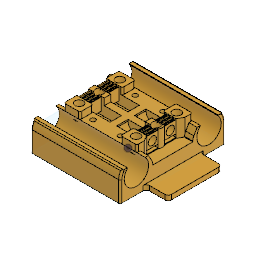
Direct_X_carriage v7 (Autodesk Fusion 360 design; units mm, degrees)
Autodesk Fusion 360 part; units mm, degrees
note: some values were not read from the file. Set by a fixed rule: which face or edge a step refers to.
sketch "スケッチ1" plane through (0, 0, 0) normal (0, 0, 1) x (1, 0, 0)
  line L0 (-27.5, 32.3) -> (27.5, 32.3)
  line L1 (27.5, 32.3) -> (27.5, 12.3)
  line L2 (27.5, 12.3) -> (18.5, 12.3)
  line L3 (18.5, 12.3) -> (18.5, -12.3)
  line L4 (18.5, -12.3) -> (27.5, -12.3)
  line L5 (27.5, -12.3) -> (27.5, -32.3)
  line L6 (27.5, -32.3) -> (-27.5, -32.3)
  line L7 (-27.5, -32.3) -> (-27.5, -12.3)
  line L8 (-27.5, -12.3) -> (-18.5, -12.3)
  line L9 (-18.5, -12.3) -> (-18.5, 12.3)
  line L10 (-18.5, 12.3) -> (-27.5, 12.3)
  line L11 (-27.5, 12.3) -> (-27.5, 32.3)
  circle A0 centre (0, 0) radius 1.75
  dimension "d1" = 55
  dimension "d2" = 64.6
  dimension "d3" = 20
  dimension "d4" = 20
  dimension "d5" = 9
  dimension "d6" = 27.5
  dimension "d7" = 32.3
  dimension "d8" = 9
  dimension "d9" = 3.5
  constraint perpendicular L0 L1
  constraint perpendicular L1 L2
  constraint perpendicular L2 L3
  constraint perpendicular L1 L4
  constraint perpendicular L4 L5
  constraint perpendicular L5 L6
  constraint perpendicular L4 L7
  constraint perpendicular L7 L8
  constraint perpendicular L8 L9
  constraint perpendicular L9 L10
  constraint perpendicular L0 L11
  constraint collinear L2 L10
  constraint collinear L4 L8
  constraint collinear L1 L5
  constraint collinear L7 L11
  constraint horizontal L0
  constraint coincident A0.centre origin
  measures "d1" horizontal distance of L5.end L6.end
  measures "d2" distance of L0 L6
  measures "d3" vertical distance of L0.end L1.end
  measures "d4" vertical distance of L4.end L5.end
  measures "d5" horizontal distance of L1.end L2.end
  measures "d6" distance of A0.centre L5
  measures "d7" distance of A0.centre L0
  measures "d8" horizontal distance of L9.end L10.end
  measures "d9" diameter of A0
extrude "押し出し1" add sketch "スケッチ1" along normal blind 17.3 makes body 1
sketch "スケッチ2" plane through (27.5, 0, 0) normal (1, 0, 0) x (0, 1, 0)
  line L0 (12.3, 0) -> (32.3, 0)
  line L1 (32.3, 0) -> (32.3, 17.3)
  line L2 (32.3, 17.3) -> (12.3, 17.3)
  line L3 (12.3, 17.3) -> (12.3, 0)
  line L4 (22.3, 0) -> (22.3, 17.3) construction
  line L5 (12.3, 12.6228) -> (32.3, 12.6228) construction
  circle A0 centre (22.3, 12) radius 7.495
  line L6 (32.3, 12.6228) -> (29.5996, 17.3)
  line L7 (32.3, 12.6228) -> (38.6199, 12.6228) construction
  line L8 (12.3, 12.6228) -> (15.0004, 17.3)
  line L9 (12.3, 17.3) -> (-12.3, 17.3)
  line L10 (0, 0) -> (0, 17.3) construction
  circle A1 centre (-22.3, 12) radius 7.495
  line L11 (-12.3, 12.6228) -> (-15.0004, 17.3)
  line L12 (-32.3, 12.6228) -> (-29.5996, 17.3)
  line L13 (-32.3, 17.3) -> (-12.3, 17.3)
  line L14 (-32.3, 0) -> (-32.3, 17.3)
  line L15 (-12.3, 17.3) -> (-12.3, 0)
  circle A2 centre (22.3, 12) radius 10.0194
  circle A3 centre (-22.3, 12) radius 10.0194
  point P0 (0, 17.3)
  dimension "d12" = 12.6228
  dimension "d13" = 14.99
  dimension "d14" = 120
  dimension "d15" = 60
  dimension "d135" = 12
  constraint midpoint L0 L4.start
  constraint midpoint L2 L4.end
  constraint coincident L3 L5.start
  constraint coincident L1 L5.end
  constraint perpendicular L1 L5
  constraint coincident L2 L6.end
  constraint horizontal L7
  constraint coincident L2 L8.end
  constraint coincident L4 A0.centre
  constraint coincident L10.start origin
  constraint coincident P0 L10.end
  constraint symmetric L5.start L10 L11.start
  constraint symmetric L5.end L10 L12.start
  constraint symmetric A0 L10 A1
  constraint symmetric L6.end L10 L12.end
  constraint symmetric L8.end L10 L11.end
  constraint symmetric L0.start L10 L15.end
  constraint symmetric L0.end L10 L14.start
  constraint symmetric L1.end L10 L13.start
  constraint symmetric L2.end L10 L9.end
  constraint concentric A0 A2
  constraint coincident L5.end A2
  constraint concentric A1 A3
  constraint coincident L12.start A3
  measures "d12" distance of L0 L5
  measures "d13" diameter of A0
  measures "d14" angle of L6 L7
  measures "d15" angle of L7 L8
  measures "d135" distance of L4.start A0.centre
extrude "押し出し2" cut sketch "スケッチ2" against normal blind 55 contours L1 L2 A2 | L2 A0 | A1 L13 | L13 L14 A3 picked at (23.4851, 8.0373) picked at (-20.2164, 11.6826) bodies 1
extrude "押し出し3" cut sketch "スケッチ2" against normal blind 9 contours L2 L8 A2 | L2 L3 A2 | L11 L13 A3 | L13 L15 A3 bodies 1
extrude "押し出し4" cut sketch "スケッチ2" against normal blind 9 from surface at -46 contours L2 L8 A2 | L2 L3 A2 | L11 L13 A3 | L13 L15 A3 bodies 1
sketch "スケッチ3" plane through (0, 0, 17.3) normal (0, 0, 1) x (-1, 0, 0)
  line L0 (18.5, -15.0004) -> (18.5, 15.0004)
  line L1 (27.5, 15.0004) -> (27.5, 17.0005)
  line L2 (-27.5, 17.0005) -> (-27.5, 15.0004)
  line L3 (-18.5, 15.0004) -> (-18.5, -15.0004)
  line L4 (-18.5, -15.0004) -> (-27.5, -15.0004)
  line L5 (-27.5, -15.0004) -> (-27.5, -17.0005)
  line L6 (-27.5, -17.0005) -> (27.5, -17.0005)
  line L7 (27.5, -17.0005) -> (27.5, -15.0004)
  line L8 (27.5, -15.0004) -> (18.5, -15.0004)
  circle A0 centre (0, 0) radius 1.75
  line L9 (-12.5, -17.0005) -> (-12.5, -9)
  line L10 (-2, -9) -> (-22.5, -9)
  line L11 (-22.5, -9) -> (-22.5, -17.0005)
  line L12 (-22.5, -17.0005) -> (-12.5, -17.0005)
  line L13 (-2, -9) -> (-2, -2)
  line L14 (-2, -2) -> (-18.5, -2)
  line L15 (27.5, 17.0005) -> (-27.5, 17.0005)
  line L16 (-27.5, 15.0004) -> (-18.5, 15.0004)
  line L17 (18.5, 15.0004) -> (27.5, 15.0004)
  dimension "d23" = 10
  dimension "d24" = 12.5
  dimension "d26" = 7
  dimension "d27" = 2
  dimension "d28" = 16.5
  constraint coincident L6 L9.start
  constraint perpendicular L6 L9
  constraint perpendicular L9 L10
  constraint coincident L6 L11.end
  constraint perpendicular L6 L11
  constraint vertical L13
  constraint coincident L3 L14.end
  constraint perpendicular L3 L14
  constraint coincident L9.end L10
  measures "d23" horizontal distance of L9.start L11.end
  measures "d24" horizontal distance of A0.centre L9.start
  measures "d26" vertical distance of L13.end L10.start
  measures "d27" distance of A0.centre L14
  measures "d28" horizontal distance of L13.end L14.end
extrude "押し出し5" cut sketch "スケッチ3" against normal blind 5.9 contours L3 L10 L13 L14 bodies 1
fillet "フィレット3" radius 5 1 edges at (2, 5.5, 11.4) on bodies 1
mirror "ミラー1" about plane through (0, 0, 0) normal (0, 1, 0) of "押し出し5", "フィレット3"
mirror "ミラー2" about plane through (0, 0, 0) normal (1, 0, 0) of "押し出し5", "フィレット3", "ミラー1"
extrude "押し出し6" add sketch "スケッチ3" against normal blind 12.3 separate body contours L3 L4 L6 L9 L10 L11 L12 | L3 L4 L10 L11 makes body 2
chamfer "面取り2" distance 4 distance2 6.4 1 edges at (22.5, 13.0002, 5) measured on face at (17.8333, 13.667, 5) on bodies 2
extrude "押し出し7" add sketch "スケッチ3" along normal blind 4.1 contours L3 L4 L6 L9 L10 L11 L12 | L3 L4 L10 L11 bodies 2
chamfer "面取り3" distance 2 distance2 3.5 1 edges at (22.5, 9, 16.4) measured on face at (15.8333, 9, 12.6) on bodies 2
sketch "スケッチ4" plane through (0, 0, 21.4) normal (0, 0, 1) x (-1, 0, 0)
  line L0 (-20.5, -9) -> (-22.5, -12.5)
  line L1 (-22.5, -12.5) -> (-22.5, -17.0005)
  line L2 (-22.5, -17.0005) -> (-12.5, -17.0005)
  line L3 (-12.5, -17.0005) -> (-12.5, -9)
  line L4 (-12.5, -9) -> (-20.5, -9)
  line L5 (-17.5, -9) -> (-17.5, -17.0005) construction
  line L6 (-22.5, -12.5) -> (-12.5, -12.5) construction
  circle A0 centre (-17.5, -12.5) radius 1.75
  circle A1 centre (-17.5, -12.5) radius 2.35
  circle A2 centre (-17.5, -12.5) radius 2.5
  dimension "d47" = 3.5
  dimension "d48" = 5
  dimension "d50" = 5
  dimension "d51" = 4.7
  dimension "d53" = 3.5
  constraint coincident L4 L5.start
  constraint coincident L2 L5.end
  constraint coincident L1 L0.end
  constraint coincident L3 L6.end
  constraint perpendicular L4 L5
  constraint perpendicular L3 L6
  constraint midpoint L6 A0.centre
  constraint concentric A0 A1
  constraint concentric A1 A2
  measures "d47" distance of L3.end L6.end
  measures "d48" distance of L1 L5
  measures "d50" diameter of A2
  measures "d51" diameter of A1
  measures "d53" diameter of A0
fillet "フィレット1" radius 1 3 edges at (12.5, 9, 13.2) (12.5, 17.0005, 13.2) (22.5, 17.0005, 16.4) on bodies 2
extrude "押し出し19" cut sketch "スケッチ2" against normal blind 20 contours L2 A0 picked at (23.4851, 8.0373) bodies 2
mirror "ミラー3" about plane through (0, 0, 0) normal (0, 1, 0) of bodies 2 makes body 3
sketch "スケッチ5" plane through (0, 9, 0) normal (0, -1, 0) x (1, 0, 0)
  line L0 (13.5, 21.4) -> (13.5, 5)
  line L1 (13.5, 5) -> (18.5, 5)
  line L2 (18.5, 5) -> (20.5, 8.2)
  line L3 (20.5, 8.2) -> (20.5, 21.4)
  line L4 (20.5, 21.4) -> (13.5, 21.4)
  line L5 (13.5, 13.4) -> (20.5, 13.4)
  line L6 (14.5, 13.4) -> (14.5, 21.4)
  line L7 (20.5, 20.95) -> (14.5, 20.95)
  line L8 (17.5, 20.95) -> (17.5, 20.2) construction
  arc A0 (17.0011, 20.5118) -> (17.9989, 20.5118) centre (17.5, 20.755) ccw
  arc A1 (16.9, 20.95) -> (17.0011, 20.5118) centre (17.9, 20.95) ccw
  arc A2 (17.9989, 20.5118) -> (18.1, 20.95) centre (17.1, 20.95) ccw
  arc A3 (15.9989, 20.5118) -> (16.1, 20.95) centre (15.1, 20.95) ccw
  arc A4 (15.0011, 20.5118) -> (15.9989, 20.5118) centre (15.5, 20.755) ccw
  arc A5 (14.9, 20.95) -> (15.0011, 20.5118) centre (15.9, 20.95) ccw
  arc A6 (19.9989, 20.5118) -> (20.1, 20.95) centre (19.1, 20.95) ccw
  arc A7 (19.0011, 20.5118) -> (19.9989, 20.5118) centre (19.5, 20.755) ccw
  arc A8 (18.9, 20.95) -> (19.0011, 20.5118) centre (19.9, 20.95) ccw
  dimension "d62" = 8
  dimension "d63" = 6
  dimension "d64" = 0.45
  dimension "d65" = 0.75
  dimension "d70" = 0.555
  dimension "d71" = 1
  dimension "d72" = 1
  dimension "d75" = 2
  dimension "d76" = 0
  constraint coincident L0 L5.start
  constraint coincident L3 L5.end
  constraint perpendicular L0 L5
  constraint coincident L5 L6.start
  constraint coincident L4 L6.end
  constraint perpendicular L5 L6
  constraint coincident L3 L7.start
  constraint coincident L6 L7.end
  constraint perpendicular L6 L7
  constraint midpoint L7 L8.start
  constraint vertical L8
  constraint coincident L8 A0.centre
  constraint coincident L7 A1.centre
  constraint coincident L7 A2.centre
  constraint coincident L7 A1.start
  constraint coincident L7 A2.end
  constraint coincident L8.end A0
  constraint tangent A0 A1
  constraint coincident A0.start A1.end
  constraint coincident A0.end A2.start
  constraint tangent A0 A2
  measures "d62" distance of L4 L5
  measures "d63" distance of L3 L6
  measures "d64" distance of L4 L7
  measures "d65" distance of L8.start L8.end
  measures "d70" radius of A0
  measures "d71" radius of A1
  measures "d72" radius of A2
extrude "押し出し11" add sketch "スケッチ5" along normal up to surface (18 mm away) contours L3 L5 L6 L7 A0 A1 A2 A3 A4 A5 A6 A7 A8 bodies 2 3
fillet "フィレット2" radius 0.0001 6 edges at (14.9, 0, 20.95) (16.1, 0, 20.95) (16.9, 0, 20.95) (18.1, 0, 20.95) (18.9, 0, 20.95) (20.1, 0, 20.95) on bodies 2
sketch "スケッチ6" plane through (0, 0, 13.4) normal (0, 0, -1) x (1, 0, 0)
  line L0 (20.5, 9) -> (14.5, 9)
  line L1 (14.5, 9) -> (14.5, -9)
  line L2 (14.5, -9) -> (20.5, -9)
  line L3 (20.5, -9) -> (20.5, 9)
  line L4 (14.5, 0) -> (20.5, 0) construction
  line L5 (14.5, 2) -> (20.5, 2)
  line L6 (14.5, -2) -> (20.5, -2)
  dimension "d87" = 2
  dimension "d88" = 2
  constraint midpoint L1 L4.start
  constraint midpoint L3 L4.end
  constraint coincident L1 L5.start
  constraint coincident L3 L5.end
  constraint perpendicular L3 L5
  constraint coincident L1 L6.start
  constraint coincident L3 L6.end
  constraint perpendicular L3 L6
  measures "d87" distance of L4 L5
  measures "d88" distance of L4 L6
extrude "押し出し15" add sketch "スケッチ6" against normal blind 8 contours L1 L3 L5 L6 bodies 2
sketch "スケッチ7" plane through (0, 0, 21.4) normal (0, 0, 1) x (-1, 0, 0)
  line L0 (-14.5, -2) -> (-14.5, 2)
  line L1 (-14.5, 2) -> (-20.5, 2)
  line L2 (-20.5, 2) -> (-20.5, -2)
  line L3 (-20.5, -2) -> (-14.5, -2)
  line L4 (-14.5, 0) -> (-20.5, 0) construction
  circle A0 centre (-17.5, 0) radius 2
  circle A1 centre (-17.5, 0) radius 2.5
  circle A2 centre (-17.5, 0) radius 2.55
  dimension "d91" = 4
  dimension "d92" = 5
  dimension "d93" = 5.1
  constraint midpoint L0 L4.start
  constraint midpoint L2 L4.end
  constraint midpoint L4 A0.centre
  constraint concentric A0 A1
  constraint concentric A1 A2
  measures "d91" diameter of A0
  measures "d92" diameter of A1
  measures "d93" diameter of A2
sketch "スケッチ8" plane through (20.5, 0, 0) normal (1, 0, 0) x (0, 1, 0)
  line L0 (-9, 13.4) -> (9, 13.4)
  line L1 (9, 13.4) -> (9, 20.95)
  line L2 (9, 20.95) -> (2, 20.95)
  line L3 (2, 20.95) -> (2, 21.4)
  line L4 (2, 21.4) -> (-2, 21.4)
  line L5 (-2, 21.4) -> (-2, 20.95)
  line L6 (-2, 20.95) -> (-9, 20.95)
  line L7 (-9, 20.95) -> (-9, 13.4)
  line L8 (9, 16.9) -> (-9, 16.9) construction
  line L9 (5.5, 13.4) -> (5.5, 20.95) construction
  circle A0 centre (5.5, 16.9) radius 2.55
  circle A1 centre (5.5, 16.9) radius 2.55
  dimension "d104" = 3.5
  dimension "d105" = 3.5
  dimension "d106" = 5.1
  dimension "d107" = 5.1
  constraint coincident L7 L8.end
  constraint coincident L0 L9.start
  constraint coincident L2 L9.end
  constraint perpendicular L2 L9
  constraint coincident L8 A0.centre
  constraint coincident L9 A0.centre
  constraint concentric A0 A1
  measures "d104" distance of L1 L9
  measures "d105" distance of L0 L8
  measures "d106" diameter of A0
  measures "d107" diameter of A1
extrude "押し出し20" cut sketch "スケッチ8" against normal blind 10 contours A0 A1 bodies 2
extrude "押し出し21" cut sketch "スケッチ8" against normal blind 0.5 contours A0 A1 bodies 2
mirror "ミラー6" about plane through (0, 0, 0) normal (0, 1, 0) of "押し出し20", "押し出し21"
mirror "ミラー5" about plane through (0, 0, 0) normal (1, 0, 0) of bodies 2 makes body 4
combine "結合1" operation add target body 1 tool bodies 2 4
sketch "スケッチ9" plane through (0, 0, 21.4) normal (0, 0, 1) x (-1, 0, 0)
  line L0 (-22.5, -12.5) -> (-22.5, -16.0005)
  arc A0 (-22.5, -16.0005) -> (-21.5, -17.0005) centre (-21.5, -16.0005) ccw
  line L1 (-21.5, -17.0005) -> (-13.5, -17.0005)
  arc A1 (-13.5, -17.0005) -> (-12.5, -16.0005) centre (-13.5, -16.0005) ccw
  line L2 (-12.5, -16.0005) -> (-12.5, -10)
  arc A2 (-12.5, -10) -> (-13.5, -9) centre (-13.5, -10) ccw
  line L3 (-13.5, -9) -> (-20.5, -9)
  line L4 (-20.5, -9) -> (-22.5, -12.5)
  line L5 (-12.5, -12.5) -> (-22.5, -12.5) construction
  line L6 (-17.5, -17.0005) -> (-17.5, -8.8071) construction
  circle A3 centre (-17.5, -12.5) radius 2
  circle A4 centre (-17.5, -12.5) radius 2.55
  circle A5 centre (-17.5, -12.5) radius 2.55
  dimension "d113" = 5
  dimension "d114" = 3.5
  dimension "d115" = 5.1
  dimension "d116" = 5.1
  dimension "d117" = 4
  constraint coincident L2 L5.start
  constraint coincident L0 L4.end
  constraint coincident L1 L6.start
  constraint perpendicular L1 L6
  constraint perpendicular L2 L5
  constraint midpoint L5 A3.centre
  constraint concentric A3 A4
  constraint concentric A4 A5
  measures "d113" distance of L2 L6
  measures "d114" distance of L3 L5
  measures "d115" diameter of A5
  measures "d116" diameter of A4
  measures "d117" diameter of A3
extrude "押し出し22" [suppressed]
extrude "押し出し23" cut sketch "スケッチ9" against normal blind 8 contours A3 | A4 A5 bodies 1
extrude "押し出し24" cut sketch "スケッチ9" against normal blind 0.5 contours A3 | A4 A5 bodies 1
mirror "ミラー7" about plane through (0, 0, 0) normal (0, 1, 0) of "押し出し23", "押し出し24"
mirror "ミラー8" about plane through (0, 0, 0) normal (1, 0, 0) of "押し出し23", "押し出し24", "ミラー7"
extrude "押し出し25" [suppressed]
extrude "押し出し26" cut sketch "スケッチ7" against normal blind 7 contours L3 A1 A2 | L1 L3 A1 A2 | L1 A1 A2 | L3 A1 | L1 L3 A0 A1 | L1 L3 A1 A2 | L1 A1 | L1 L3 A0 A1 | A0 bodies 1
extrude "押し出し27" [suppressed]
mirror "ミラー9" about plane through (0, 0, 0) normal (1, 0, 0) of "押し出し26"
fillet "フィレット4" radius 5 6 edges at (0, 32.3, 12.6228) (24.9429, 12.3, 12.6228) (-24.9429, 12.3, 12.6228) (0, -32.3, 12.6228) (24.9429, -12.3, 12.6228) (-24.9429, -12.3, 12.6228) on bodies 1
fillet "フィレット5" radius 1 10 edges at (27.5, 32.3, 6.3114) (-27.5, 32.3, 6.3114) (-27.5, -32.3, 6.3114) (27.5, -32.3, 6.3114) (27.5, 31.8424, 15.0546) (-27.5, 31.8424, 15.0546) (0, 30.8028, 17.3) (27.5, -31.8424, 15.0546) (-27.5, -31.8424, 15.0546) (0, -30.8028, 17.3) on bodies 1
chamfer "Chamfer6" distance 0.4 angle 45 2 edges at (0, -27.5995, 17.3) (0, 27.5995, 17.3) on bodies 1
sketch "スケッチ10" plane through (0, 0, 0) normal (0, 0, -1) x (1, 0, 0)
  circle A0 centre (0, 0) radius 1.75
  line L0 (27.5, 12.3) -> (27.5, 31.3)
  arc A1 (27.5, 31.3) -> (26.5, 32.3) centre (26.5, 31.3) ccw
  line L1 (26.5, 32.3) -> (-26.5, 32.3)
  arc A2 (-26.5, 32.3) -> (-27.5, 31.3) centre (-26.5, 31.3) ccw
  line L2 (-27.5, 31.3) -> (-27.5, 12.3)
  line L3 (-27.5, 12.3) -> (-18.5, 12.3)
  line L4 (-18.5, 12.3) -> (-18.5, -12.3)
  line L5 (-18.5, -12.3) -> (-27.5, -12.3)
  line L6 (-27.5, -12.3) -> (-27.5, -31.3)
  arc A3 (-27.5, -31.3) -> (-26.5, -32.3) centre (-26.5, -31.3) ccw
  line L7 (-26.5, -32.3) -> (26.5, -32.3)
  arc A4 (26.5, -32.3) -> (27.5, -31.3) centre (26.5, -31.3) ccw
  line L8 (27.5, -31.3) -> (27.5, -12.3)
  line L9 (27.5, -12.3) -> (18.5, -12.3)
  line L10 (18.5, -12.3) -> (18.5, 12.3)
  line L11 (18.5, 12.3) -> (27.5, 12.3)
  circle A5 centre (12, 12) radius 1.525
  circle A6 centre (-12, 12) radius 1.525
  circle A7 centre (-12, -12) radius 1.525
  circle A8 centre (12, -12) radius 1.525
  dimension "d139" = 3.05
  dimension "d140" = 12
  dimension "d141" = 12
  dimension "d143" = 360
  measures "d139" diameter of A5
  measures "d140" horizontal distance of A0.centre A5.centre
  measures "d141" vertical distance of A0.centre A5.centre
extrude "押し出し28" [suppressed]
sketch "Sketch39" plane through (0, 0, 17.3) normal (0, 0, 1) x (-1, 0, 0)
  circle A0 centre (0, 0) radius 1.75
  line L0 (14.5, -2) -> (14.5, 2)
  line L1 (14.5, 2) -> (2, 2)
  line L2 (2, 2) -> (2, 9)
  line L3 (2, 9) -> (13.5, 9)
  arc A1 (12.5, 10) -> (13.5, 9) centre (13.5, 10) ccw
  line L4 (12.5, 10) -> (12.5, 16.0005)
  arc A2 (13.5, 17.0005) -> (12.5, 16.0005) centre (13.5, 16.0005) ccw
  line L5 (13.5, 17.0005) -> (-13.5, 17.0005)
  arc A3 (-12.5, 16.0005) -> (-13.5, 17.0005) centre (-13.5, 16.0005) ccw
  line L6 (-12.5, 16.0005) -> (-12.5, 10)
  arc A4 (-13.5, 9) -> (-12.5, 10) centre (-13.5, 10) ccw
  line L7 (-13.5, 9) -> (-2, 9)
  line L8 (-2, 9) -> (-2, 2)
  line L9 (-2, 2) -> (-14.5, 2)
  line L10 (-14.5, 2) -> (-14.5, -2)
  line L11 (-14.5, -2) -> (-2, -2)
  line L12 (-2, -2) -> (-2, -9)
  line L13 (-2, -9) -> (-13.5, -9)
  arc A5 (-12.5, -10) -> (-13.5, -9) centre (-13.5, -10) ccw
  line L14 (-12.5, -10) -> (-12.5, -16.0005)
  arc A6 (-13.5, -17.0005) -> (-12.5, -16.0005) centre (-13.5, -16.0005) ccw
  line L15 (-13.5, -17.0005) -> (13.5, -17.0005)
  arc A7 (12.5, -16.0005) -> (13.5, -17.0005) centre (13.5, -16.0005) ccw
  line L16 (12.5, -16.0005) -> (12.5, -10)
  arc A8 (13.5, -9) -> (12.5, -10) centre (13.5, -10) ccw
  line L17 (13.5, -9) -> (2, -9)
  line L18 (2, -9) -> (2, -2)
  line L19 (2, -2) -> (14.5, -2)
  line L20 (12.5, -13.0002) -> (-12.5, -13.0002) construction
  line L21 (12.5, 13.0002) -> (-12.5, 13.0002) construction
  line L22 (-8.5, 13.0002) -> (8.5, 13.0002) construction
  line L23 (8.5, 13.0002) -> (8.5, -13.0002) construction
  line L24 (8.5, -13.0002) -> (-8.5, -13.0002) construction
  line L25 (-8.5, -13.0002) -> (-8.5, 13.0002) construction
  line L26 (-8.5, 13.0002) -> (8.5, -13.0002) construction
  line L27 (8.5, 13.0002) -> (-8.5, -13.0002) construction
  circle A9 centre (-8.5, -13.0002) radius 1.5
  circle A10 centre (8.5, -13.0002) radius 1.5
  circle A11 centre (8.5, 13.0002) radius 1.5
  circle A12 centre (-8.5, 13.0002) radius 1.5
  dimension "d210" = 8.5
  dimension "d211" = 3
  dimension "d212" = 3
  dimension "d213" = 3
  dimension "d214" = 3
  constraint midpoint L16 L20.start
  constraint midpoint L14 L20.end
  constraint midpoint L4 L21.start
  constraint midpoint L6 L21.end
  constraint perpendicular L22 L23
  constraint parallel L22 L24
  constraint parallel L23 L25
  constraint horizontal L22
  constraint coincident L26 A0.centre
  constraint coincident L27 A0.centre
  constraint coincident A0.centre origin
  constraint collinear L21 L22
  constraint coincident L24.end L25.start
  constraint coincident L23.end L24.start
  constraint coincident L22.end L23.start
  constraint coincident L22.start L25.end
  measures "d210" distance of A0.centre L25
  measures "d211" diameter of A9
  measures "d212" diameter of A10
  measures "d213" diameter of A11
  measures "d214" diameter of A12
extrude "Extrude53" cut sketch "Sketch39" against normal through all contours A9 | A10 | A11 | A12 bodies 1
sketch "Sketch12" plane through (0, 0, 13.4) normal (0, 0, -1) x (1, 0, 0)
  line L0 (18.5, -2) -> (14.5, -2)
  line L1 (14.5, -2) -> (14.5, -9)
  line L2 (14.5, -9) -> (20.5, -9)
  line L3 (20.5, -9) -> (20.5, 9)
  line L4 (20.5, 9) -> (14.5, 9)
  line L5 (14.5, 9) -> (14.5, 2)
  line L6 (14.5, 2) -> (18.5, 2)
  line L7 (18.5, 2) -> (18.5, -2)
  line L8 (-14.5, -2) -> (-18.5, -2)
  line L9 (-18.5, -2) -> (-18.5, 2)
  line L10 (-18.5, 2) -> (-14.5, 2)
  line L11 (-14.5, 2) -> (-14.5, 9)
  line L12 (-14.5, 9) -> (-20.5, 9)
  line L13 (-20.5, 9) -> (-20.5, -9)
  line L14 (-20.5, -9) -> (-14.5, -9)
  line L15 (-14.5, -9) -> (-14.5, -2)
  line L16 (18.5, 2) -> (20.5, 2)
  line L17 (20.5, 2) -> (20.5, -2)
  line L18 (20.5, -2) -> (18.5, -2)
  line L19 (18.5, -2) -> (18.5, 2)
  line L20 (-18.5, 2) -> (-20.5, 2)
  line L21 (-20.5, 2) -> (-20.5, -2)
  line L22 (-20.5, -2) -> (-18.5, -2)
  line L23 (-18.5, -2) -> (-18.5, 2)
  point P0 (20.5, -2)
  point P1 (-20.5, -2)
  constraint horizontal L16
  constraint vertical L17
  constraint horizontal L18
  constraint vertical L19
  constraint coincident P0 L17.end
  constraint coincident L6.end L7.start
  constraint horizontal L20
  constraint vertical L21
  constraint horizontal L22
  constraint vertical L23
  constraint coincident P1 L21.end
  constraint coincident L9.end L10.start
extrude "Extrude29" add sketch "Sketch12" along normal blind 5 contours L3 L7 L16 L17 L18 L19 bodies 1
sketch "Sketch14" plane through (0, 2, 0) normal (0, 1, 0) x (-1, 0, 0)
  line L0 (-14.5, 13.4) -> (-20.5, 13.4)
  line L1 (-20.5, 13.4) -> (-20.5, 8.4)
  line L2 (-20.5, 8.4) -> (-18.5, 8.4)
  line L3 (-18.5, 8.4) -> (-18.5, 11.4)
  line L4 (-18.5, 11.4) -> (-7, 11.4)
  arc A0 (-7, 11.4) -> (-2, 16.4) centre (-7, 16.4) ccw
  line L5 (-2, 16.4) -> (-2, 17.3)
  line L6 (-2, 17.3) -> (-14.5, 17.3)
  line L7 (-14.5, 17.3) -> (-14.5, 13.4)
  line L8 (-20.5, 13.4) -> (-20.5, 8.2)
  line L9 (-18.5, 11.4) -> (-18.5, 5)
  line L10 (-20.5, 8.4) -> (-18.5, 8.4)
  line L11 (-18.5, 11.4) -> (-20.5, 11.4)
  line L12 (-20.5, 11.4) -> (-20.5, 8.4)
  line L13 (-20.5, 8.4) -> (-18.5, 8.4)
  line L14 (-18.5, 8.4) -> (-18.5, 11.4)
  point P0 (-18.5, 11.4)
  point P1 (-20.5, 8.4)
  constraint horizontal L11
  constraint vertical L12
  constraint horizontal L13
  constraint vertical L14
  constraint coincident P1 L1.end
  constraint coincident P0 L3.end
extrude "Extrude31" add sketch "Sketch14" along normal up to surface (-11 mm away) and the other way up to surface (-7 mm away) contours L1 L2 L3 L8 L9 L10 L11 L12 L13 L14 bodies 1
chamfer "Chamfer4" distance 2.5 distance2 2 1 edges at (20.5, 0, 8.4) measured on face at (20.5, 0.6667, 9.4) on bodies 1
mirror "Mirror10" about plane through (0, 0, 0) normal (1, 0, 0) of "Extrude29", "Extrude31", "Chamfer4"
sketch "Sketch15" plane through (0, 0, 21.4) normal (0, 0, 1) x (-1, 0, 0)
  line L0 (22.5, -12.5) -> (20.5, -9)
  line L1 (20.5, -9) -> (13.5, -9)
  arc A0 (13.5, -9) -> (12.5, -10) centre (13.5, -10) ccw
  line L2 (12.5, -10) -> (12.5, -16.0005)
  arc A1 (12.5, -16.0005) -> (13.5, -17.0005) centre (13.5, -16.0005) ccw
  line L3 (13.5, -17.0005) -> (21.5, -17.0005)
  arc A2 (21.5, -17.0005) -> (22.5, -16.0005) centre (21.5, -16.0005) ccw
  line L4 (22.5, -16.0005) -> (22.5, -12.5)
  line L5 (-11, -18) -> (-25, -18)
  line L6 (-25, -18) -> (-25, 19)
  line L7 (-25, 19) -> (-11, 19)
  line L8 (-11, 19) -> (-11, -18)
  circle A3 centre (17.5, -12.5) radius 2.55
  constraint horizontal L5
  constraint vertical L6
  constraint horizontal L7
  constraint vertical L8
sketch "Sketch16" plane through (0, 0, 17.3) normal (0, 0, 1) x (-1, 0, 0)
  circle A0 centre (0, 0) radius 1.75
  line L0 (14.5, -2) -> (14.5, 2)
  line L1 (14.5, 2) -> (2, 2)
  line L2 (2, 2) -> (2, 9)
  line L3 (2, 9) -> (13.5, 9)
  arc A1 (12.5, 10) -> (13.5, 9) centre (13.5, 10) ccw
  line L4 (12.5, 10) -> (12.5, 16.0005)
  arc A2 (13.5, 17.0005) -> (12.5, 16.0005) centre (13.5, 16.0005) ccw
  line L5 (13.5, 17.0005) -> (-13.5, 17.0005)
  arc A3 (-12.5, 16.0005) -> (-13.5, 17.0005) centre (-13.5, 16.0005) ccw
  line L6 (-12.5, 16.0005) -> (-12.5, 10)
  arc A4 (-13.5, 9) -> (-12.5, 10) centre (-13.5, 10) ccw
  line L7 (-13.5, 9) -> (-2, 9)
  line L8 (-2, 9) -> (-2, 2)
  line L9 (-2, 2) -> (-14.5, 2)
  line L10 (-14.5, 2) -> (-14.5, -2)
  line L11 (-14.5, -2) -> (-2, -2)
  line L12 (-2, -2) -> (-2, -9)
  line L13 (-2, -9) -> (-13.5, -9)
  arc A5 (-12.5, -10) -> (-13.5, -9) centre (-13.5, -10) ccw
  line L14 (-12.5, -10) -> (-12.5, -16.0005)
  arc A6 (-13.5, -17.0005) -> (-12.5, -16.0005) centre (-13.5, -16.0005) ccw
  line L15 (-13.5, -17.0005) -> (13.5, -17.0005)
  arc A7 (12.5, -16.0005) -> (13.5, -17.0005) centre (13.5, -16.0005) ccw
  line L16 (12.5, -16.0005) -> (12.5, -10)
  arc A8 (13.5, -9) -> (12.5, -10) centre (13.5, -10) ccw
  line L17 (13.5, -9) -> (2, -9)
  line L18 (2, -9) -> (2, -2)
  line L19 (2, -2) -> (14.5, -2)
  line L20 (-14.5, -2) -> (-12.5712, -2)
  line L21 (-12.5712, -2) -> (-12.5712, 2)
  line L22 (-12.5712, 2) -> (-14.5, 2)
  line L23 (-14.5, 2) -> (-14.5, -2)
  circle A9 centre (-8.5, -13.0002) radius 1.5
  circle A10 centre (-8.5, 13.0002) radius 1.5
  circle A11 centre (8.5, -13.0002) radius 1.5
  circle A12 centre (8.5, 13.0002) radius 1.5
  constraint horizontal L20
  constraint vertical L21
  constraint horizontal L22
  constraint vertical L23
  constraint coincident L9 L21.end
  constraint coincident L10.end L11.start
extrude "Extrude33" add sketch "Sketch16" along normal up to surface (4.1 mm away) contours L9 L10 L11 L20 L21 L22 L23 bodies 1
mirror "Mirror11" about plane through (0, 0, 0) normal (1, 0, 0) of "Extrude33"
sketch "Sketch22" plane through (18.5, 0, 0) normal (1, 0, 0) x (0, 1, 0)
  line L0 (9, 8.4) -> (-9, 8.4)
  line L1 (-9, 8.4) -> (-9, 5)
  line L2 (-9, 5) -> (-12.3, 5)
  line L3 (-12.3, 5) -> (-12.3, 0)
  line L4 (-12.3, 0) -> (12.3, 0)
  line L5 (12.3, 0) -> (12.3, 5)
  line L6 (12.3, 5) -> (9, 5)
  line L7 (9, 5) -> (9, 8.4)
  line L8 (-12.3, 0) -> (12.3, 0)
  line L9 (12.3, 0) -> (12.3, 10.9)
  line L10 (12.3, 10.9) -> (-12.3, 10.9)
  line L11 (-12.3, 10.9) -> (-12.3, 0)
  line L12 (-9, 10.9) -> (9, 10.9)
  constraint horizontal L8
  constraint vertical L9
  constraint horizontal L10
  constraint vertical L11
  constraint coincident L9.end L12
  constraint coincident L3.end L4.start
  constraint collinear L5 L9
extrude "Extrude37" add sketch "Sketch22" along normal up to surface (9 mm away) bodies 1
sketch "Sketch23" plane through (-18.5, 0, 0) normal (-1, 0, 0) x (0, -1, 0)
  line L0 (9, 8.4) -> (-9, 8.4)
  line L1 (-9, 8.4) -> (-9, 5)
  line L2 (-9, 5) -> (-12.3, 5)
  line L3 (-12.3, 5) -> (-12.3, 0)
  line L4 (-12.3, 0) -> (12.3, 0)
  line L5 (12.3, 0) -> (12.3, 5)
  line L6 (12.3, 5) -> (9, 5)
  line L7 (9, 5) -> (9, 8.4)
  line L8 (-12.3, 0) -> (12.3, 0)
  line L9 (12.3, 0) -> (12.3, 10.9)
  line L10 (12.3, 10.9) -> (-12.3, 10.9)
  line L11 (-12.3, 10.9) -> (-12.3, 0)
  line L12 (9, 10.9) -> (-9, 10.9)
  constraint horizontal L8
  constraint vertical L9
  constraint horizontal L10
  constraint vertical L11
  constraint coincident L9.end L12
  constraint coincident L3.end L4.start
  constraint collinear L5 L9
extrude "Extrude38" add sketch "Sketch23" along normal up to surface (9 mm away) bodies 1
fillet "Fillet7" [suppressed]
sketch "Sketch25" plane through (0, 0, 21.4) normal (0, 0, 1) x (-1, 0, 0)
  arc A0 (-19.0819, 2) -> (-19.0819, -2) centre (-17.5, 0) ccw
  line L0 (-19.0819, 2) -> (-20.5, 2)
  line L1 (-20.5, 2) -> (-20.5, -2)
  line L2 (-20.5, -2) -> (-19.0819, -2)
  circle A1 centre (-17.5, 0) radius 3.6056
  constraint concentric A0 A1
  constraint coincident L1.end A1
extrude "Extrude40" add sketch "Sketch25" against normal up to surface (10.5 mm away) contours L1 A1 bodies 1
sketch "Sketch26" plane through (0, 0, 21.4) normal (0, 0, 1) x (-1, 0, 0)
  arc A0 (19.0819, -2) -> (19.0819, 2) centre (17.5, 0) ccw
  line L0 (19.0819, -2) -> (20.5, -2)
  line L1 (20.5, -2) -> (20.5, 2)
  line L2 (20.5, 2) -> (19.0819, 2)
  circle A1 centre (17.5, 0) radius 3.6056
  constraint concentric A0 A1
  constraint coincident L0.end A1
extrude "Extrude41" add sketch "Sketch26" against normal up to surface (10.5 mm away) contours L1 A1 bodies 1
chamfer "Chamfer5" distance 4.9 angle 45 1 edges at (27.5, 0, 10.9) on bodies 1
sketch "Sketch27" plane through (20.5, 0, 0) normal (1, 0, 0) x (0, 1, 0)
  circle A0 centre (-5.5, 16.9) radius 2.55
  line L0 (-2, 13.4) -> (-2, 20.95)
  line L1 (-2, 20.95) -> (-9, 20.95)
  line L2 (-9, 20.95) -> (-9, 13.4)
  line L3 (-9, 13.4) -> (-2, 13.4)
extrude "Extrude42" add sketch "Sketch27" against normal up to surface (6 mm away) contours A0 bodies 1
sketch "Sketch28" plane through (20.5, 0, 0) normal (1, 0, 0) x (0, 1, 0)
  line L0 (2, 20.95) -> (2, 13.4)
  line L1 (2, 13.4) -> (9, 13.4)
  line L2 (9, 13.4) -> (9, 20.95)
  line L3 (9, 20.95) -> (2, 20.95)
  circle A0 centre (5.5, 16.9) radius 2.55
extrude "Extrude43" add sketch "Sketch28" against normal up to surface (6 mm away) contours A0 bodies 1
sketch "Sketch29" plane through (20.5, 0, 0) normal (1, 0, 0) x (0, 1, 0)
  line L0 (-2, 13.4) -> (-2, 20.95)
  line L1 (-2, 20.95) -> (-9, 20.95)
  line L2 (-9, 20.95) -> (-9, 13.4)
  line L3 (-9, 13.4) -> (-2, 13.4)
  line L4 (-2.0613, 20.5118) -> (-9, 20.5118)
  line L5 (-12.5, 20.5118) -> (12.5, 20.5118)
  line L6 (12.5, 20.5118) -> (12.5, 10.9)
  line L7 (12.5, 10.9) -> (-12.5, 10.9)
  line L8 (-12.5, 10.9) -> (-12.5, 20.5118)
  line L9 (-2, 10.9) -> (-9, 10.9)
  line L10 (-12.5, 12.6831) -> (-12.5, 21.4)
  line L11 (12.5, 12.6831) -> (12.5, 21.4)
  constraint horizontal L5
  constraint vertical L6
  constraint horizontal L7
  constraint vertical L8
  constraint collinear L4 L5
  constraint collinear L7 L9
  constraint collinear L8 L10
  constraint collinear L6 L11
extrude "Extrude44" add sketch "Sketch29" along normal up to surface (2 mm away) contours L0 L2 L3 L4 L5 | L0 L2 L3 L5 L6 L7 L8 L9 L10 L11 bodies 1
sketch "Sketch30" plane through (0, 0, 20.5118) normal (0, 0, 1) x (-1, 0, 0)
  line L0 (-22.5, -12.5) -> (-20.5, -9)
  line L1 (-20.5, -9) -> (-20.5, -2)
  arc A0 (-20.5, 2) -> (-20.5, -2) centre (-17.5, 0) ccw
  line L2 (-20.5, 2) -> (-20.5, 9)
  line L3 (-20.5, 9) -> (-22.5, 12.5)
  line L4 (-22.5, 12.5) -> (-22.5, -12.5)
  line L5 (-20.5, -2) -> (-22.5, -2)
  line L6 (-22.5, -2) -> (-22.5, 2)
  line L7 (-22.5, 2) -> (-20.5, 2)
  line L8 (-20.5, 2) -> (-20.5, -2)
  line L9 (-19.0819, 2) -> (-20.5, 2)
  constraint horizontal L5
  constraint vertical L6
  constraint horizontal L7
  constraint vertical L8
  constraint coincident L4 L6.end
  constraint coincident L1.end A0.end
  constraint collinear L7 L9
extrude "Extrude45" add sketch "Sketch30" along normal up to surface (0.8882 mm away) contours A0 L4 L5 L6 L7 bodies 1
sketch "Sketch31" plane through (0, 0, 20.5118) normal (0, 0, 1) x (-1, 0, 0)
  line L0 (-22.5, 2) -> (-20.5, 2)
  line L1 (-20.5, 2) -> (-20.5, 9)
  line L2 (-20.5, 9) -> (-22.5, 12.5)
  line L3 (-22.5, 12.5) -> (-22.5, 2)
  line L4 (-20.5, 9) -> (-22.5, 9)
  constraint coincident L1.end L2.start
  constraint coincident L3 L4.end
  constraint perpendicular L3 L4
extrude "Extrude46" add sketch "Sketch31" along normal up to surface (0.8882 mm away) contours L2 L3 L4 bodies 1
sketch "Sketch32" plane through (0, 0, 20.5118) normal (0, 0, 1) x (-1, 0, 0)
  line L0 (-20.5, -2) -> (-22.5, -2)
  line L1 (-22.5, -2) -> (-22.5, -12.5)
  line L2 (-22.5, -12.5) -> (-20.5, -9)
  line L3 (-20.5, -9) -> (-20.5, -2)
  line L4 (-20.5, -9) -> (-22.5, -9)
  constraint coincident L2.end L3.start
  constraint coincident L1 L4.end
  constraint perpendicular L1 L4
extrude "Extrude47" add sketch "Sketch32" along normal up to surface (0.8882 mm away) contours L1 L2 L4 bodies 1
sketch "Sketch33" plane through (0, 0, 20.95) normal (0, 0, 1) x (-1, 0, 0)
  line L0 (-20.1001, -2) -> (-20.5, -2)
  line L1 (-20.5, -2) -> (-20.5, -9)
  line L2 (-20.5, -9) -> (-20.1001, -9)
  line L3 (-20.1001, -9) -> (-20.1001, -2)
  line L4 (-27.5, -31.3) -> (-27.5, 31.3)
  arc A0 (-26.5, 32.3) -> (-27.5, 31.3) centre (-26.5, 31.3) ccw
  line L5 (-26.5, 32.3) -> (26.5, 32.3)
  arc A1 (27.5, 31.3) -> (26.5, 32.3) centre (26.5, 31.3) ccw
  arc A2 (26.5, -32.3) -> (27.5, -31.3) centre (26.5, -31.3) ccw
  line L6 (26.5, -32.3) -> (-26.5, -32.3)
  arc A3 (-27.5, -31.3) -> (-26.5, -32.3) centre (-26.5, -31.3) ccw
  line L7 (27.5, 31.3) -> (27.5, -31.3)
  circle A4 centre (0, 0) radius 1.75
  circle A5 centre (-8.5, -13.0002) radius 1.5
  circle A6 centre (-8.5, 13.0002) radius 1.5
  circle A7 centre (8.5, -13.0002) radius 1.5
  circle A8 centre (8.5, 13.0002) radius 1.5
sketch "Sketch34" plane through (0, 0, 20.95) normal (0, 0, 1) x (-1, 0, 0)
  line L0 (-20.9001, -2) -> (-20.1001, -2)
  line L1 (-20.1001, -2) -> (-20.1001, -9)
  line L2 (-20.1001, -9) -> (-20.9001, -9)
  line L3 (-20.9001, -9) -> (-20.9001, -2)
  line L4 (-20.1001, -2) -> (-20.1001, -9)
  line L5 (-13.5, -9) -> (-22.5, -9)
  line L6 (-19.0819, -2) -> (-22.5, -2)
  dimension "d199" = 0.8
  constraint horizontal L0
  constraint vertical L1
  constraint horizontal L2
  constraint vertical L3
  constraint coincident L1.end L4
  constraint collinear L2 L5
  constraint collinear L0 L6
  measures "d199" distance of L0.start L0.end
extrude "Extrude48" add sketch "Sketch34" against normal up to surface (0.4382 mm away) bodies 1
sketch "Sketch35" plane through (0, 0, 20.95) normal (0, 0, 1) x (-1, 0, 0)
sketch "Sketch36" plane through (0, 0, 20.95) normal (0, 0, 1) x (-1, 0, 0)
sketch "Sketch37" plane through (0, 0, 20.95) normal (0, 0, 1) x (-1, 0, 0)
sketch "Sketch38" plane through (0, 0, 20.95) normal (0, 0, 1) x (-1, 0, 0)
  line L0 (-20.9001, 9) -> (-20.1001, 9)
  line L1 (-20.1001, 9) -> (-20.1001, 2)
  line L2 (-20.1001, 2) -> (-20.9001, 2)
  line L3 (-20.9001, 2) -> (-20.9001, 9)
  line L4 (-20.1001, 9) -> (-20.1001, 2)
  line L5 (-19.0819, 2) -> (-22.5, 2)
  line L6 (-13.5, 9) -> (-22.5, 9)
  dimension "d202" = 0.8
  constraint horizontal L0
  constraint vertical L1
  constraint horizontal L2
  constraint vertical L3
  constraint coincident L1.end L4
  constraint collinear L2 L5
  constraint collinear L0 L6
  measures "d202" distance of L1 L3
extrude "Extrude49" add sketch "Sketch38" against normal up to surface (0.4382 mm away) bodies 1
extrude "Extrude50" cut 2 faces at (21.4334, -2.0409, 20.5118) (21.9667, -4.3742, 20.5118) along direction (0, 0, -1) blind 0.3 on bodies 1 bodies 1
extrude "Extrude51" cut 1 faces at (21.9667, 6.6667, 20.5118) along direction (0, 0, -1) blind 0.3 on bodies 1 bodies 1
extrude "Extrude52" cut 2 faces at (20.5, 6.6667, 12.0667) (20.5, -6.6667, 12.7333) along direction (1, 0, 0) through all on bodies 1 bodies 1
extrude "Extrude54" add sketch "スケッチ1" along normal up to surface (17.3 mm away) contours A0 bodies 1
sketch "Sketch42" plane through (0, 0, 0) normal (0, 0, -1) x (1, 0, 0)
  circle A0 centre (8.5, -13.0002) radius 1.5
  circle A1 centre (8.5, 13.0002) radius 1.5
  circle A2 centre (-8.5, -13.0002) radius 1.5
  circle A3 centre (-8.5, 13.0002) radius 1.5
  arc A4 (27.5, 31.3) -> (26.5, 32.3) centre (26.5, 31.3) ccw
  line L0 (26.5, 32.3) -> (-26.5, 32.3)
  arc A5 (-26.5, 32.3) -> (-27.5, 31.3) centre (-26.5, 31.3) ccw
  line L1 (-27.5, 31.3) -> (-27.5, -31.3)
  arc A6 (-27.5, -31.3) -> (-26.5, -32.3) centre (-26.5, -31.3) ccw
  line L2 (-26.5, -32.3) -> (26.5, -32.3)
  arc A7 (26.5, -32.3) -> (27.5, -31.3) centre (26.5, -31.3) ccw
  line L3 (27.5, -31.3) -> (27.5, 31.3)
  line L4 (-27.5, -16.3) -> (-41, -16.3)
  line L5 (-41, -16.3) -> (-41, 16.7)
  line L6 (-41, 16.7) -> (-27.5, 16.7)
  line L7 (-27.5, 16.7) -> (-27.5, -16.3)
  dimension "d227" = 13.5
  dimension "d228" = 16
  dimension "d229" = 33
  constraint horizontal L4
  constraint vertical L5
  constraint horizontal L6
  constraint vertical L7
  constraint coincident L1 L4.start
  measures "d227" distance of L5.end L6.end
  measures "d228" distance of L2 L4
  measures "d229" distance of L4.end L5.end
extrude "Extrude57" add sketch "Sketch42" against normal blind 3 contours L1 L4 L5 L6 L7 bodies 1
fillet "Fillet9" radius 2 4 edges at (-27.5, 16.3, 1.5) (-41, 16.3, 1.5) (-41, -16.7, 1.5) (-27.5, -16.7, 1.5) on bodies 1
sketch "Sketch43" plane through (0, 0, 0) normal (0, 0, -1) x (1, 0, 0)
  circle A0 centre (8.5, -13.0002) radius 1.5
  circle A1 centre (8.5, 13.0002) radius 1.5
  circle A2 centre (-8.5, -13.0002) radius 1.5
  circle A3 centre (-8.5, 13.0002) radius 1.5
  arc A4 (-39, 16.7) -> (-41, 14.7) centre (-39, 14.7) ccw
  line L0 (-41, 14.7) -> (-41, -14.3)
  arc A5 (-41, -14.3) -> (-39, -16.3) centre (-39, -14.3) ccw
  line L1 (-39, -16.3) -> (-29.5, -16.3)
  arc A6 (-27.5, -18.3) -> (-29.5, -16.3) centre (-29.5, -18.3) ccw
  line L2 (-27.5, -18.3) -> (-27.5, -31.3)
  arc A7 (-27.5, -31.3) -> (-26.5, -32.3) centre (-26.5, -31.3) ccw
  line L3 (-26.5, -32.3) -> (26.5, -32.3)
  arc A8 (26.5, -32.3) -> (27.5, -31.3) centre (26.5, -31.3) ccw
  line L4 (27.5, -31.3) -> (27.5, 31.3)
  arc A9 (27.5, 31.3) -> (26.5, 32.3) centre (26.5, 31.3) ccw
  line L5 (26.5, 32.3) -> (-26.5, 32.3)
  arc A10 (-26.5, 32.3) -> (-27.5, 31.3) centre (-26.5, 31.3) ccw
  line L6 (-27.5, 31.3) -> (-27.5, 18.7)
  arc A11 (-29.5, 16.7) -> (-27.5, 18.7) centre (-29.5, 18.7) ccw
  line L7 (-29.5, 16.7) -> (-39, 16.7)
move_body "Move1" bodies 1 to x (-1, 0, 0) y (0, -1, 0) z (0, 0, 1) at (0, 0, 0)
equation "d2 = 65 mm - 0.4 mm"
equation "d6 = d1 / 2"
equation "d7 = d2 / 2"
equation "d8 = d5"
equation "d91 = 3.5 mm + 0.5 mm"
equation "d92 = 4.7 mm + 0.3 mm"
equation "d93 = 5 mm + 0.1 mm"
equation "d106 = 5 mm + 0.1 mm"
equation "d107 = 4.7 mm + 0.4 mm"
equation "d115 = 5 mm + 0.1 mm"
equation "d116 = 4.7 mm + 0.4 mm"
equation "d117 = 3.5 mm + 0.5 mm"
equation "d212 = d211"
equation "d213 = d211"
equation "d214 = d211"
